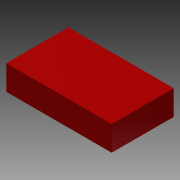
# Autodesk Inventor part: rbc
Saved by Autodesk Inventor 2015 SP1 (Build 190203100, 203)
## iProperties
Created: 2015-04-20
Part Number: rbc
Material: Ogólny
Document SubType Name: Modeling
Designer: Marcin
Density: 1 g/cm^3
Appearance: Gładkie - czerwone
Author: Marcin
Autodesk Inventor part; units mm, degrees
ref_plane "YZ Plane" through (0, 0, 0) normal (1, 0, 0) x (0, 1, 0)
ref_plane "XZ Plane" through (0, 0, 0) normal (0, 1, 0) x (-1, 0, 0)
ref_plane "XY Plane" through (0, 0, 0) normal (0, 0, 1) x (1, 0, 0)
sketch "Szkic1" plane through (0, 0, 0) normal (0, 0, 1) x (1, 0, 0)
  line L0 (-42.5, -25) -> (42.5, -25)
  line L1 (42.5, -25) -> (42.5, 25)
  line L2 (42.5, 25) -> (-42.5, 25)
  line L3 (-42.5, 25) -> (-42.5, -25)
  line L4 (-42.5, -25) -> (42.5, 25) construction
  line L5 (42.5, -25) -> (-42.5, 25) construction
  point P0 (0, 0)
  dimension "d0" = 85
  dimension "d1" = 50
  constraints: 12 end point, 2 midpoint, 2 parallel, 1 horizontal, 1 perpendicular
  measures "d0" distance of L1.end L2.end
  measures "d1" distance of L0.end L1.end
extrude "Wyciągnięcie proste1" add sketch "Szkic1" along normal mid plane 20
